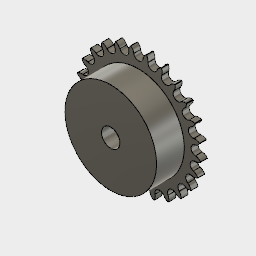
Chain Guide Assembly (Autodesk Fusion 360 archive; units mm, degrees)
design "1/4  25T Sprocket"
Autodesk Fusion 360 part; units mm, degrees
sketch "Sketch1" plane through (0, 0, 0) normal (0, 0, 1) x (1, 0, 0)
  circle A0 centre (0, 0) radius 19.875
  circle A1 centre (0, 0) radius 4
  circle A2 centre (0, 0) radius 27 construction
  line L0 (0, 27) -> (0, -27) construction
  line L1 (0, 24.875) -> (6.1862, 24.0935) construction
  line L2 (3.0931, 24.4843) -> (0, 0) construction
  line L3 (3.0931, 24.4843) -> (3.384, 26.7871) construction
  line L4 (3.384, 26.7871) -> (3.2848, 26.7996)
  line L5 (3.384, 26.7871) -> (3.4832, 26.7746)
  arc A3 (3.2848, 26.7996) -> (1.9842, 24.6243) centre (5.1153, 24.2288) ccw
  arc A4 (4.2019, 24.3442) -> (3.4832, 26.7746) centre (1.0709, 24.7397) ccw
  arc A5 (-1.9842, 24.6243) -> (1.9842, 24.6243) centre (0, 24.875) ccw
  line L6 (-6.1862, 24.0935) -> (0, 24.875) construction
  line L7 (-3.0931, 24.4843) -> (-3.384, 26.7871) construction
  line L8 (-3.384, 26.7871) -> (-3.2848, 26.7996)
  line L9 (-3.384, 26.7871) -> (-3.4832, 26.7746)
  arc A6 (-8.0457, 23.3573) -> (-4.2019, 24.3442) centre (-6.1862, 24.0935) ccw
  arc A7 (-1.9842, 24.6243) -> (-3.2848, 26.7996) centre (-5.1153, 24.2288) ccw
  arc A8 (-3.4832, 26.7746) -> (-4.2019, 24.3442) centre (-1.0709, 24.7397) ccw
  line L10 (-11.9836, 21.7981) -> (-6.1862, 24.0935) construction
  line L11 (-9.0849, 22.9458) -> (-9.9394, 25.104) construction
  line L12 (-9.9394, 25.104) -> (-9.8464, 25.1408)
  line L13 (-9.9394, 25.104) -> (-10.0323, 25.0672)
  arc A9 (-13.6017, 20.6226) -> (-10.1241, 22.5344) centre (-11.9836, 21.7981) ccw
  arc A10 (-8.0457, 23.3573) -> (-9.8464, 25.1408) centre (-10.98, 22.1955) ccw
  arc A11 (-10.0323, 25.0672) -> (-10.1241, 22.5344) centre (-7.1898, 23.6962) ccw
  line L14 (-17.0281, 18.1331) -> (-11.9836, 21.7981) construction
  line L15 (-14.5059, 19.9656) -> (-15.8702, 21.8435) construction
  line L16 (-15.8702, 21.8435) -> (-15.7893, 21.9022)
  line L17 (-15.8702, 21.8435) -> (-15.9511, 21.7847)
  arc A12 (-18.303, 16.5921) -> (-15.4101, 19.3087) centre (-17.0281, 18.1331) ccw
  arc A13 (-13.6017, 20.6226) -> (-15.7893, 21.9022) centre (-16.1549, 18.7675) ccw
  arc A14 (-15.9511, 21.7847) -> (-15.4101, 19.3087) centre (-12.8569, 21.1637) ccw
  line L18 (-21.0027, 13.3287) -> (-17.0281, 18.1331) construction
  line L19 (-19.0154, 15.7309) -> (-20.8039, 17.2104) construction
  line L20 (-20.8039, 17.2104) -> (-20.7401, 17.2875)
  line L21 (-20.8039, 17.2104) -> (-20.8676, 17.1334)
  arc A15 (-21.8542, 11.519) -> (-19.7278, 14.8697) centre (-21.0027, 13.3287) ccw
  arc A16 (-18.303, 16.5921) -> (-20.7401, 17.2875) centre (-20.3146, 14.1604) ccw
  arc A17 (-20.8676, 17.1334) -> (-19.7278, 14.8697) centre (-17.7161, 17.3014) ccw
  line L22 (-23.6575, 7.6868) -> (-21.0027, 13.3287) construction
  line L23 (-22.3301, 10.5077) -> (-24.4303, 11.496) construction
  line L24 (-24.4303, 11.496) -> (-24.3878, 11.5865)
  line L25 (-24.4303, 11.496) -> (-24.4729, 11.4056)
  arc A18 (-24.0323, 5.7222) -> (-22.806, 9.4965) centre (-23.6575, 7.6868) ccw
  arc A19 (-21.8542, 11.519) -> (-24.3878, 11.5865) centre (-23.1979, 8.6635) ccw
  arc A20 (-24.4729, 11.4056) -> (-22.806, 9.4965) centre (-21.4622, 12.352) ccw
  line L26 (-24.8259, 1.5619) -> (-23.6575, 7.6868) construction
  line L27 (-24.2417, 4.6244) -> (-26.5218, 5.0593) construction
  line L28 (-26.5218, 5.0593) -> (-26.503, 5.1575)
  line L29 (-26.5218, 5.0593) -> (-26.5405, 4.9611)
  arc A21 (-24.7003, -0.4341) -> (-24.4512, 3.5265) centre (-24.8259, 1.5619) ccw
  arc A22 (-24.0323, 5.7222) -> (-26.503, 5.1575) centre (-24.6237, 2.6222) ccw
  arc A23 (-26.5405, 4.9611) -> (-24.4512, 3.5265) centre (-23.8598, 6.6265) ccw
  line L30 (-24.4344, -4.6611) -> (-24.8259, 1.5619) construction
  line L31 (-24.6302, -1.5496) -> (-26.9467, -1.6953) construction
  line L32 (-26.9467, -1.6953) -> (-26.953, -1.5955)
  line L33 (-26.9467, -1.6953) -> (-26.9404, -1.7951)
  arc A24 (-23.8164, -6.5632) -> (-24.56, -2.6651) centre (-24.4344, -4.6611) ccw
  arc A25 (-24.7003, -0.4341) -> (-26.953, -1.5955) centre (-24.5022, -3.5838) ccw
  arc A26 (-26.9404, -1.7951) -> (-24.56, -2.6651) centre (-24.7581, 0.4847) ccw
  line L34 (-22.5076, -10.5913) -> (-24.4344, -4.6611) construction
  line L35 (-23.471, -7.6262) -> (-25.6785, -8.3435) construction
  line L36 (-25.6785, -8.3435) -> (-25.7094, -8.2484)
  line L37 (-25.6785, -8.3435) -> (-25.6476, -8.4386)
  arc A27 (-21.4359, -12.2799) -> (-23.1256, -8.6891) centre (-22.5076, -10.5913) ccw
  arc A28 (-23.8164, -6.5632) -> (-25.7094, -8.2484) centre (-22.8411, -9.5647) ccw
  arc A29 (-25.6476, -8.4386) -> (-23.1256, -8.6891) centre (-24.1008, -5.6877) ccw
  line L38 (-19.1665, -15.8559) -> (-22.5076, -10.5913) construction
  line L39 (-20.837, -13.2236) -> (-22.7969, -14.4673) construction
  line L40 (-22.7969, -14.4673) -> (-22.8504, -14.3829)
  line L41 (-22.7969, -14.4673) -> (-22.7433, -14.5518)
  arc A30 (-17.7086, -17.225) -> (-20.2382, -14.1673) centre (-19.1665, -15.8559) ccw
  arc A31 (-21.4359, -12.2799) -> (-22.8504, -14.3829) centre (-19.7449, -14.9446) ccw
  arc A32 (-22.7433, -14.5518) -> (-20.2382, -14.1673) centre (-21.9292, -11.5026) ccw
  line L42 (-14.6212, -20.1243) -> (-19.1665, -15.8559) construction
  line L43 (-16.8938, -17.9901) -> (-18.4828, -19.6822) construction
  line L44 (-18.4828, -19.6822) -> (-18.5557, -19.6137)
  line L45 (-18.4828, -19.6822) -> (-18.4099, -19.7506)
  arc A33 (-12.8685, -21.0878) -> (-16.0791, -18.7552) centre (-14.6212, -20.1243) ccw
  arc A34 (-17.7086, -17.225) -> (-18.5557, -19.6137) centre (-15.408, -19.3854) ccw
  arc A35 (-18.4099, -19.7506) -> (-16.0791, -18.7552) centre (-18.3797, -16.5948) ccw
  line L46 (-9.1571, -23.1282) -> (-14.6212, -20.1243) construction
  line L47 (-11.8891, -21.6262) -> (-13.0073, -23.6603) construction
  line L48 (-13.0073, -23.6603) -> (-13.095, -23.6121)
  line L49 (-13.0073, -23.6603) -> (-12.9197, -23.7085)
  arc A36 (-7.2199, -23.6256) -> (-10.9097, -22.1647) centre (-9.1571, -23.1282) ccw
  arc A37 (-12.8685, -21.0878) -> (-13.095, -23.6121) centre (-10.103, -22.6082) ccw
  arc A38 (-12.9197, -23.7085) -> (-10.9097, -22.1647) centre (-13.6753, -20.6443) ccw
  line L50 (-3.1177, -24.6789) -> (-9.1571, -23.1282) construction
  line L51 (-6.1374, -23.9035) -> (-6.7146, -26.1517) construction
  line L52 (-6.7146, -26.1517) -> (-6.8115, -26.1269)
  line L53 (-6.7146, -26.1517) -> (-6.6178, -26.1766)
  arc A39 (-1.1177, -24.6789) -> (-5.0548, -24.1815) centre (-3.1177, -24.6789) ccw
  arc A40 (-7.2199, -23.6256) -> (-6.8115, -26.1269) centre (-4.1631, -24.4104) ccw
  arc A41 (-6.6178, -26.1766) -> (-5.0548, -24.1815) centre (-8.1116, -23.3966) ccw
  line L54 (3.1177, -24.6789) -> (-3.1177, -24.6789) construction
  line L55 (0, -24.6789) -> (0, -27) construction
  line L56 (0, -27) -> (-0.1, -27)
  line L57 (0, -27) -> (0.1, -27)
  arc A42 (5.0548, -24.1815) -> (1.1177, -24.6789) centre (3.1177, -24.6789) ccw
  arc A43 (-1.1177, -24.6789) -> (-0.1, -27) centre (2.0383, -24.6789) ccw
  arc A44 (0.1, -27) -> (1.1177, -24.6789) centre (-2.0383, -24.6789) ccw
  line L58 (9.1571, -23.1282) -> (3.1177, -24.6789) construction
  line L59 (6.1374, -23.9035) -> (6.7146, -26.1517) construction
  line L60 (6.7146, -26.1517) -> (6.6178, -26.1766)
  line L61 (6.7146, -26.1517) -> (6.8115, -26.1269)
  arc A45 (10.9097, -22.1647) -> (7.2199, -23.6256) centre (9.1571, -23.1282) ccw
  arc A46 (5.0548, -24.1815) -> (6.6178, -26.1766) centre (8.1116, -23.3966) ccw
  arc A47 (6.8115, -26.1269) -> (7.2199, -23.6256) centre (4.1631, -24.4104) ccw
  line L62 (14.6212, -20.1243) -> (9.1571, -23.1282) construction
  line L63 (11.8891, -21.6262) -> (13.0073, -23.6603) construction
  line L64 (13.0073, -23.6603) -> (12.9197, -23.7085)
  line L65 (13.0073, -23.6603) -> (13.095, -23.6121)
  arc A48 (16.0791, -18.7552) -> (12.8685, -21.0878) centre (14.6212, -20.1243) ccw
  arc A49 (10.9097, -22.1647) -> (12.9197, -23.7085) centre (13.6753, -20.6443) ccw
  arc A50 (13.095, -23.6121) -> (12.8685, -21.0878) centre (10.103, -22.6082) ccw
  line L66 (19.1665, -15.8559) -> (14.6212, -20.1243) construction
  line L67 (16.8938, -17.9901) -> (18.4828, -19.6822) construction
  line L68 (18.4828, -19.6822) -> (18.4099, -19.7506)
  line L69 (18.4828, -19.6822) -> (18.5557, -19.6137)
  arc A51 (20.2382, -14.1673) -> (17.7086, -17.225) centre (19.1665, -15.8559) ccw
  arc A52 (16.0791, -18.7552) -> (18.4099, -19.7506) centre (18.3797, -16.5948) ccw
  arc A53 (18.5557, -19.6137) -> (17.7086, -17.225) centre (15.408, -19.3854) ccw
  line L70 (22.5076, -10.5913) -> (19.1665, -15.8559) construction
  line L71 (20.837, -13.2236) -> (22.7969, -14.4673) construction
  line L72 (22.7969, -14.4673) -> (22.7433, -14.5518)
  line L73 (22.7969, -14.4673) -> (22.8504, -14.3829)
  arc A54 (23.1256, -8.6891) -> (21.4359, -12.2799) centre (22.5076, -10.5913) ccw
  arc A55 (20.2382, -14.1673) -> (22.7433, -14.5518) centre (21.9292, -11.5026) ccw
  arc A56 (22.8504, -14.3829) -> (21.4359, -12.2799) centre (19.7449, -14.9446) ccw
  line L74 (24.4344, -4.6611) -> (22.5076, -10.5913) construction
  line L75 (23.471, -7.6262) -> (25.6785, -8.3435) construction
  line L76 (25.6785, -8.3435) -> (25.6476, -8.4386)
  line L77 (25.6785, -8.3435) -> (25.7094, -8.2484)
  arc A57 (24.56, -2.6651) -> (23.8164, -6.5632) centre (24.4344, -4.6611) ccw
  arc A58 (23.1256, -8.6891) -> (25.6476, -8.4386) centre (24.1008, -5.6877) ccw
  arc A59 (25.7094, -8.2484) -> (23.8164, -6.5632) centre (22.8411, -9.5647) ccw
  line L78 (24.8259, 1.5619) -> (24.4344, -4.6611) construction
  line L79 (24.6302, -1.5496) -> (26.9467, -1.6953) construction
  line L80 (26.9467, -1.6953) -> (26.9404, -1.7951)
  line L81 (26.9467, -1.6953) -> (26.953, -1.5955)
  arc A60 (24.4512, 3.5265) -> (24.7003, -0.4341) centre (24.8259, 1.5619) ccw
  arc A61 (24.56, -2.6651) -> (26.9404, -1.7951) centre (24.7581, 0.4847) ccw
  arc A62 (26.953, -1.5955) -> (24.7003, -0.4341) centre (24.5022, -3.5838) ccw
  line L82 (23.6575, 7.6868) -> (24.8259, 1.5619) construction
  line L83 (24.2417, 4.6244) -> (26.5218, 5.0593) construction
  line L84 (26.5218, 5.0593) -> (26.5405, 4.9611)
  line L85 (26.5218, 5.0593) -> (26.503, 5.1575)
  arc A63 (22.806, 9.4965) -> (24.0323, 5.7222) centre (23.6575, 7.6868) ccw
  arc A64 (24.4512, 3.5265) -> (26.5405, 4.9611) centre (23.8598, 6.6265) ccw
  arc A65 (26.503, 5.1575) -> (24.0323, 5.7222) centre (24.6237, 2.6222) ccw
  line L86 (21.0027, 13.3287) -> (23.6575, 7.6868) construction
  line L87 (22.3301, 10.5077) -> (24.4303, 11.496) construction
  line L88 (24.4303, 11.496) -> (24.4729, 11.4056)
  line L89 (24.4303, 11.496) -> (24.3878, 11.5865)
  arc A66 (19.7278, 14.8697) -> (21.8542, 11.519) centre (21.0027, 13.3287) ccw
  arc A67 (22.806, 9.4965) -> (24.4729, 11.4056) centre (21.4622, 12.352) ccw
  arc A68 (24.3878, 11.5865) -> (21.8542, 11.519) centre (23.1979, 8.6635) ccw
  line L90 (17.0281, 18.1331) -> (21.0027, 13.3287) construction
  line L91 (19.0154, 15.7309) -> (20.8039, 17.2104) construction
  line L92 (20.8039, 17.2104) -> (20.8676, 17.1334)
  line L93 (20.8039, 17.2104) -> (20.7401, 17.2875)
  arc A69 (15.4101, 19.3087) -> (18.303, 16.5921) centre (17.0281, 18.1331) ccw
  arc A70 (19.7278, 14.8697) -> (20.8676, 17.1334) centre (17.7161, 17.3014) ccw
  arc A71 (20.7401, 17.2875) -> (18.303, 16.5921) centre (20.3146, 14.1604) ccw
  line L94 (11.9836, 21.7981) -> (17.0281, 18.1331) construction
  line L95 (14.5059, 19.9656) -> (15.8702, 21.8435) construction
  line L96 (15.8702, 21.8435) -> (15.9511, 21.7847)
  line L97 (15.8702, 21.8435) -> (15.7893, 21.9022)
  arc A72 (10.1241, 22.5344) -> (13.6017, 20.6226) centre (11.9836, 21.7981) ccw
  arc A73 (15.4101, 19.3087) -> (15.9511, 21.7847) centre (12.8569, 21.1637) ccw
  arc A74 (15.7893, 21.9022) -> (13.6017, 20.6226) centre (16.1549, 18.7675) ccw
  line L98 (6.1862, 24.0935) -> (11.9836, 21.7981) construction
  line L99 (9.0849, 22.9458) -> (9.9394, 25.104) construction
  line L100 (9.9394, 25.104) -> (10.0323, 25.0672)
  line L101 (9.9394, 25.104) -> (9.8464, 25.1408)
  arc A75 (4.2019, 24.3442) -> (8.0457, 23.3573) centre (6.1862, 24.0935) ccw
  arc A76 (10.1241, 22.5344) -> (10.0323, 25.0672) centre (7.1898, 23.6962) ccw
  arc A77 (9.8464, 25.1408) -> (8.0457, 23.3573) centre (10.98, 22.1955) ccw
  point P0 (-6.7146, 26.1517)
  point P1 (-13.0073, 23.6603)
  point P2 (-18.4828, 19.6822)
  point P3 (-22.7969, 14.4673)
  point P4 (-25.6785, 8.3435)
  point P5 (-26.9467, 1.6953)
  point P6 (-26.5218, -5.0593)
  point P7 (-24.4303, -11.496)
  point P8 (-20.8039, -17.2104)
  point P9 (-15.8702, -21.8435)
  point P10 (-9.9394, -25.104)
  point P11 (-3.384, -26.7871)
  point P12 (3.384, -26.7871)
  point P13 (9.9394, -25.104)
  point P14 (15.8702, -21.8435)
  point P15 (20.8039, -17.2104)
  point P16 (24.4303, -11.496)
  point P17 (26.5218, -5.0593)
  point P18 (26.9467, 1.6953)
  point P19 (25.6785, 8.3435)
  point P20 (22.7969, 14.4673)
  point P21 (18.4828, 19.6822)
  point P22 (13.0073, 23.6603)
  point P23 (6.7146, 26.1517)
  dimension "d1" = 39.75
  dimension "d2" = 8
  dimension "d3" = 54
  dimension "d4" = 4
  dimension "d5" = 24.875
  dimension "d8" = 0.1
  dimension "d9" = 0.1
  dimension "d13" = 360
  measures "d1" diameter of A0
  measures "d2" diameter of A1
  measures "d3" diameter of A2
  measures "d4" diameter of A5
  measures "d5" distance of A0.centre L1.start
  measures "d8" distance of L3.end L4.end
  measures "d9" distance of L3.end L5.end
extrude "Extrude1" add sketch "Sketch1" along normal blind 3 contours A0 | L4 L5 A3 A4 A5 L8 L9 A6 A7 A8 L12 L13 A9 A10 A11 L16 L17 A12 A13 A14 L20 L21 A15 A16 A17 L24 L25 A18 A19 A20 L28 L29 A21 A22 A23 L32 L33 A24 A25 A26 L36 L37 A27 A28 A29 L40 L41 A30 A31 A32 L44 L45 A33 A34 A35 L48 L49 A36 A37 A38 L52 L53 A39 A40 A41 L56 L57 A42 A43 A44 L60 L61 A45 A46 A47 L64 L65 A48 A49 A50 L68 L69 A51 A52 A53 L72 L73 A54 A55 A56 L76 L77 A57 A58 A59 L80 L81 A60 A61 A62 L84 L85 A63 A64 A65 L88 L89 A66 A67 A68 L92 L93 A69 A70 A71 L96 L97 A72 A73 A74 L100 L101 A75 A76 A77
extrude "Extrude2" add sketch "Sketch1" along normal blind 15 contours A0
